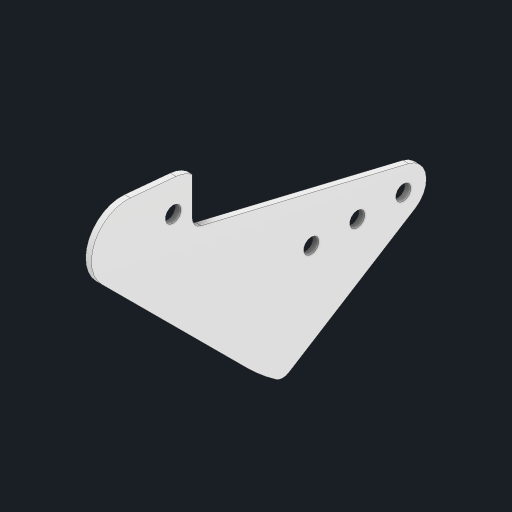
# Autodesk Inventor part: sled
Saved by Autodesk Inventor 2024 (Build 280153000, 153)
## iProperties
Created: 2024-03-23
Part Number: sled
Material: Acetal Resin, White
Document SubType Name: Modeling
Designer: Averey Ku
Density: 1.425 g/cm^3
Appearance: Smooth - White
d0: 0.165 in
d1: 0.165 in
d3: 0.125 in
d4: 0.165 in
d11: 0.125 in
Author: Averey Ku
Autodesk Inventor part; units mm, degrees
ref_plane "YZ Plane" through (0, 0, 0) normal (1, 0, 0) x (0, 1, 0)
ref_plane "XZ Plane" through (0, 0, 0) normal (0, 1, 0) x (-1, 0, 0)
ref_plane "XY Plane" through (0, 0, 0) normal (0, 0, 1) x (1, 0, 0)
sketch "main" plane through (0, 0, 0) normal (0, 0, 1) x (1, 0, 0)
  circle A0 centre (10.9635, 21.0817) radius 2.1
  circle A1 centre (10.9635, 21.0817) radius 2.0955
  arc A2 (31.3634, 3.4082) -> (38.0738, 11.3874) centre (-11.9899, 46.6796) ccw
  arc A3 (38.0738, 11.3874) -> (38.1719, 14.8984) centre (35.4788, 13.2167) ccw
  circle A4 centre (10.9635, 46.4817) radius 2.0955
  arc A5 (16.3496, 49.845) -> (4.7897, 47.9673) centre (10.9635, 46.4817) ccw
  line L0 (38.1719, 14.8984) -> (16.3496, 49.845)
  arc A6 (-25.4047, -28.8165) -> (-8.6396, -36.6705) centre (-15.6049, -29.7183) ccw
  line L1 (-8.6396, -36.6705) -> (31.3634, 3.4082)
  line L2 (-25.4047, -28.8165) -> (-24.2459, -16.2232)
  circle A7 centre (10.9635, 33.7817) radius 2.0955
  circle A8 centre (-15.6049, -17.0183) radius 2.1844
  arc A9 (-22.5138, -11.768) -> (-24.2459, -16.2232) centre (-15.6049, -17.0183) ccw
  line L3 (4.7897, 47.9673) -> (-8.9994, -9.3358)
  line L4 (-22.5138, -11.768) -> (-12.0863, -11.768)
  arc A10 (-12.0863, -11.768) -> (-8.9994, -9.3358) centre (-12.0863, -8.593) ccw
  point P0 (5.2874, 13.8034)
  point P1 (39.2673, 13.1442)
  dimension "d0" = 4.191
  dimension "d1" = 4.191
  dimension "d3" = 3.175
  dimension "d4" = 4.191
  dimension "d11" = 3.175
  measures "d0" diameter of A4
  measures "d1" diameter of A1
  measures "d3" radius of A3
  measures "d4" diameter of A7
  measures "d11" radius of A10
sketch "Sketch1" plane through (0, 0, 0) normal (1, 0, 0) x (0, 1, 0)
  circle A0 centre (0, 25.4) radius 2.1
  circle A1 centre (0, 25.4) radius 2.0955
  arc A2 (-20.3999, 43.0735) -> (-27.1104, 35.0943) centre (22.9534, -0.1979) ccw
  arc A3 (-27.1104, 35.0943) -> (-27.2084, 31.5833) centre (-24.5154, 33.265) ccw
  circle A4 centre (0, 0) radius 2.0955
  arc A5 (-5.3861, -3.3633) -> (6.1738, -1.4856) centre (0, 0) ccw
  line L0 (-27.2084, 31.5833) -> (-5.3861, -3.3633)
  arc A6 (36.3681, 75.2982) -> (19.603, 83.1522) centre (26.5684, 76.2) ccw
  line L1 (19.603, 83.1522) -> (-20.3999, 43.0735)
  line L2 (36.3681, 75.2982) -> (35.2093, 62.7049)
  circle A7 centre (0, 12.7) radius 2.0955
  circle A8 centre (26.5684, 63.5) radius 2.1844
  arc A9 (33.4773, 58.2497) -> (35.2093, 62.7049) centre (26.5684, 63.5) ccw
  line L3 (6.1738, -1.4856) -> (19.9628, 55.8175)
  line L4 (33.4773, 58.2497) -> (23.0497, 58.2497)
  arc A10 (23.0497, 58.2497) -> (19.9628, 55.8175) centre (23.0497, 55.0747) ccw
  point P0 (0, 0)
extrude "Extrusion1" add sketch "Sketch1" along normal blind 1.5875 contours L1 A6 L2 A9 L4 A10 L3 A5 L0 A3 A2
body "Solid1"
